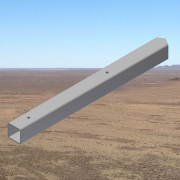
# Autodesk Inventor part: 2f2ax2
Saved by Autodesk Inventor 2014 SP1 (Build 180222100, 222)
## iProperties
Company: HERA Project
Created: 2013-06-27
Part Number: 2f2ax2
Material: Steel
Description: Feed backplane support interior piece 2
Document SubType Name: Modeling
Designer: David DeBoer
Mass: 176.671 g
Surface Area: 275.636 cm^2
Volume: 22.5058 cm^3
Density: 7.85 g/cm^3
Appearance: Steel
Title: Feed backplane support interior piece 2
Author: David DeBoer
Autodesk Inventor part; units mm, degrees
ref_plane "YZ Plane" through (0, 0, 0) normal (1, 0, 0) x (0, 1, 0)
ref_plane "XZ Plane" through (0, 0, 0) normal (0, 1, 0) x (-1, 0, 0)
ref_plane "XY Plane" through (0, 0, 0) normal (0, 0, 1) x (1, 0, 0)
sketch "Sketch1" plane through (0, 0, 0) normal (0, 0, 1) x (1, 0, 0)
  line L0 (3.7363, 0) -> (22.7863, 0)
  line L1 (25.9613, 3.175) -> (25.9613, 22.225)
  line L2 (22.7863, 25.4) -> (3.7363, 25.4)
  line L3 (0.5613, 22.225) -> (0.5613, 3.175)
  arc A0 (3.7363, 25.4) -> (0.5613, 22.225) centre (3.7363, 22.225) ccw
  arc A1 (0.5613, 3.175) -> (3.7363, 0) centre (3.7363, 3.175) ccw
  arc A2 (22.7863, 0) -> (25.9613, 3.175) centre (22.7863, 3.175) ccw
  arc A3 (25.9613, 22.225) -> (22.7863, 25.4) centre (22.7863, 22.225) ccw
  line L4 (3.7363, 23.4) -> (22.7863, 23.4)
  arc A4 (23.9613, 22.225) -> (22.7863, 23.4) centre (22.7863, 22.225) ccw
  line L5 (23.9613, 22.225) -> (23.9613, 3.175)
  arc A5 (22.7863, 2) -> (23.9613, 3.175) centre (22.7863, 3.175) ccw
  line L6 (22.7863, 2) -> (3.7363, 2)
  arc A6 (2.5613, 3.175) -> (3.7363, 2) centre (3.7363, 3.175) ccw
  line L7 (2.5613, 3.175) -> (2.5613, 22.225)
  arc A7 (3.7363, 23.4) -> (2.5613, 22.225) centre (3.7363, 22.225) ccw
  point P0 (0, 0)
  point P1 (0.5613, 0)
  point P2 (25.9613, 0)
  point P3 (0.5613, 25.4)
  dimension "d0" = 25.4
  dimension "d2" = 25.4
  dimension "d3" = 3.175
  dimension "d4" = 2
  constraints: 16 end point, 16 point on circle, 8 centre point, 8 tangent, 6 point on line, 4 parallel, 3 equal radius, 2 perpendicular, 1 horizontal, 7 other
  measures "d0" distance of point (0.561, 0) point (25.961, 0)
  measures "d2" distance of point (0.561, 25.4) point (0.561, 0)
  measures "d3" radius of A0
  measures "d4" distance between parallel lines of L4 L2
extrude "tube" add sketch "Sketch1" along normal blind 330.1
sketch "Sketch7" plane through (3.7363, 25.4, 0) normal (0, 1, 0) x (1, 0, 0)
  line L0 (19.05, 0) -> (0, 0) projected
  circle A0 centre (9.525, -25.4) radius 3.5758
  point P0 (-3.7363, 0)
  dimension "d45" = 25.4
  constraints: 1 centre point
  measures "d45" distance from line of A0.centre L0
hole "centerHole_cutOff" at (13.2613, 25.4, 25.4) direction (0, -1, 0) diameter 6.35 end through all
sketch "Sketch8" plane through (3.7363, 25.4, 0) normal (0, 1, 0) x (1, 0, 0)
  circle A0 centre (9.525, -25.4) radius 3.175 projected
  line L0 (0, 0) -> (0, -330.1) projected
  circle A1 centre (9.525, -152.4) radius 1.4483
  circle A2 centre (9.525, -302.4) radius 1.4483
  point P0 (-3.7363, 0)
  dimension "d55" = 150
  dimension "d60" = 127
  constraints: 2 centre point, 1 vertical, 2 other
  measures "d55" distance of A1.centre A2.centre
  measures "d60" distance of A1.centre A0.centre
hole "armHoles" at (13.2613, 25.4, 152.4) at (13.2613, 25.4, 302.4) direction (0, -1, 0) diameter 4.5 end through all clearance for "Flat Head Machine Screw" size "M4" standard "Ansi Metric M Profile"
sketch "Sketch9" plane through (3.7363, 25.4, 0) normal (0, 1, 0) x (1, 0, 0)
  circle A0 centre (9.525, -25.4) radius 3.175 construction
  line L0 (9.525, -25.4) -> (9.525, -40.0812) construction
  line L1 (-12.1249, -52.4308) -> (9.525, -39.9312)
  line L2 (-8.8213, -52.7845) -> (41.9787, -52.7845) construction
  line L3 (9.525, -40.0812) -> (40.882, -40.0812) construction
  line L4 (9.2652, -40.0812) -> (31.8692, -53.1316)
  line L5 (-12.1249, -52.4308) -> (-12.1249, 11.2848)
  line L6 (31.8692, -53.1316) -> (31.8692, 11.2848)
  line L7 (-12.1249, 11.2848) -> (31.8692, 11.2848)
  point P0 (-3.7363, 0)
  dimension "d68" = 14.6812
  dimension "d70" = 30
  constraints: 16 end point, 2 parallel, 2 perpendicular, 2 point on line, 1 horizontal
  measures "d68" distance of L0.start L0.end
  measures "d70" angle of L2 L1
extrude "Extrusion4" cut sketch "Sketch9" against normal blind 50.8
body "Solid1"
